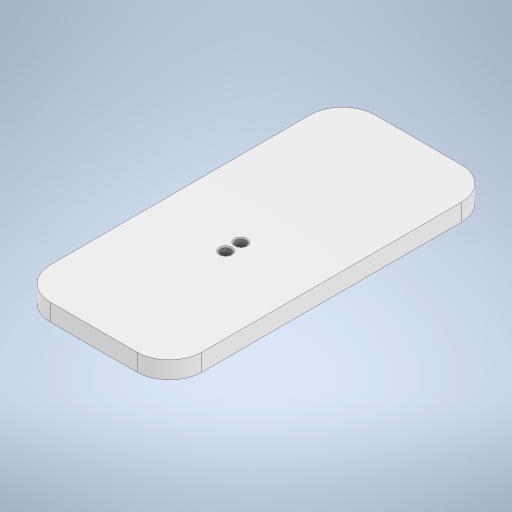
# Autodesk Inventor part: Base superior(suporte)
Saved by Autodesk Inventor 2023 (Build 270158000, 158)
## iProperties
Created: 2023-03-09
Part Number: Base superior(suporte)
Material: ABS plástico
Document SubType Name: Modeling
Designer: Antonio Ribeiro
Density: 1.06 g/cm^3
Appearance: Suave - Branco
Author: Antonio Ribeiro
Autodesk Inventor part; units mm, degrees
ref_plane "YZ Plane" through (0, 0, 0) normal (1, 0, 0) x (0, 1, 0)
ref_plane "XZ Plane" through (0, 0, 0) normal (0, 1, 0) x (-1, 0, 0)
ref_plane "XY Plane" through (0, 0, 0) normal (0, 0, 1) x (1, 0, 0)
sketch "Esboço4" plane through (0, 0, 0) normal (0, 1, 0) x (-1, 0, 0)
  line L0 (0, -15) -> (0, -135)
  line L1 (-15, -150) -> (-55, -150)
  line L2 (-70, -135) -> (-70, -15)
  line L3 (-55, 0) -> (-15, 0)
  arc A0 (-15, -150) -> (0, -135) centre (-15, -135) ccw
  arc A1 (-70, -135) -> (-55, -150) centre (-55, -135) ccw
  arc A2 (-55, 0) -> (-70, -15) centre (-55, -15) ccw
  arc A3 (0, -15) -> (-15, 0) centre (-15, -15) ccw
  point P0 (0, 0)
  point P1 (0, -150)
  point P2 (-70, -150)
  dimension "d7" = 150
  dimension "d8" = 70
  dimension "d9" = 15
  constraints: 8 end point, 8 point on circle, 8 tangent, 6 point on line, 4 centre point, 3 equal radius, 3 perpendicular, 1 vertical
  measures "d7" distance of point (0, 0) point (0, -150)
  measures "d8" distance of point (0, -150) point (-70, -150)
  measures "d9" radius of A0
extrude "Extrusão2" add sketch "Esboço4" along normal blind 8
sketch "Esboço5" plane through (0, 8, 0) normal (0, 1, 0) x (1, 0, 0)
  line L0 (15, 0) -> (55, 0) projected
  line L1 (55, 150) -> (15, 150) projected
  circle A0 centre (35, 61) radius 2.5
  circle A1 centre (35, 68) radius 2.5
  point P0 (0, 0)
  constraints: 2 centre point
extrude "Extrusão3" cut sketch "Esboço5" against normal through all
sketch "Sketch7" plane through (0, 0, 0) normal (0, -1, 0) x (1, 0, 0)
  circle A0 centre (35, -61) radius 2 projected
  circle A1 centre (35, -68) radius 2 projected
  line L0 (43, -68) -> (43, -74.75)
  line L1 (43, -74.75) -> (27, -74.75)
  line L2 (27, -74.75) -> (27, -54.25)
  line L3 (27, -54.25) -> (43, -54.25)
  line L4 (43, -54.25) -> (43, -68)
  point P0 (0, 0)
  dimension "d25" = 8
  constraints: 10 end point, 4 perpendicular, 1 point on line
  measures "d25" distance of A1.centre L0.start
extrude "Extrusion4" add sketch "Sketch7" along normal blind 10
fillet "Fillet4" radius 2 8 edges at (43, -5, -54.25) (43, -5, -74.75) (43, -10, -64.5) (35, -10, -54.25) (27, -10, -64.5) (35, -10, -74.75) (27, -5, -74.75) (27, -5, -54.25)
fillet "Fillet5" radius 0.5 2 edges at (32.5, 8, -61) (32.5, 8, -68)
